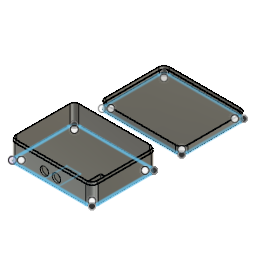
design2 (Autodesk Fusion 360 design; units mm, degrees)
Autodesk Fusion 360 part; units mm, degrees
sketch "Sketch1" plane through (0, 0, 0) normal (0, 0, 1) x (1, 0, 0)
  line L0 (10, 0) -> (170, 0)
  line L1 (180, 10) -> (180, 130)
  line L2 (170, 140) -> (10, 140)
  line L3 (0, 130) -> (0, 10)
  arc A0 (10, 140) -> (0, 130) centre (10, 130) ccw
  arc A1 (0, 10) -> (10, 0) centre (10, 10) ccw
  arc A2 (170, 0) -> (180, 10) centre (170, 10) ccw
  arc A3 (180, 130) -> (170, 140) centre (170, 130) ccw
  arc A4 (180, 130) -> (170, 140) centre (170, 130) ccw
  arc A5 (170, 0) -> (180, 10) centre (170, 10) ccw
  line L4 (-4, 130) -> (-4, 10)
  arc A6 (-4, 10) -> (10, -4) centre (10, 10) ccw
  line L5 (10, -4) -> (170, -4)
  arc A7 (170, -4) -> (184, 10) centre (170, 10) ccw
  line L6 (184, 10) -> (184, 130)
  arc A8 (184, 130) -> (170, 144) centre (170, 130) ccw
  line L7 (170, 144) -> (10, 144)
  arc A9 (10, 144) -> (-4, 130) centre (10, 130) ccw
  line L8 (-2, 130) -> (-2, 10)
  arc A10 (-2, 10) -> (10, -2) centre (10, 10) ccw
  line L9 (10, -2) -> (170, -2)
  arc A11 (170, -2) -> (182, 10) centre (170, 10) ccw
  line L10 (182, 10) -> (182, 130)
  arc A12 (182, 130) -> (170, 142) centre (170, 130) ccw
  line L11 (170, 142) -> (10, 142)
  arc A13 (10, 142) -> (-2, 130) centre (10, 130) ccw
  arc A14 (10, 142) -> (-2, 130) centre (10, 130) ccw
  arc A15 (170, -2) -> (182, 10) centre (170, 10) ccw
  line L12 (0, 130) -> (0, 10)
  line L13 (10, -4) -> (170, -4)
  arc A16 (170, 0) -> (180, 10) centre (170, 10) ccw
  line L14 (-4, 130) -> (-4, 10)
  line L15 (170, 144) -> (10, 144)
  arc A17 (184, 130) -> (170, 144) centre (170, 130) ccw
  arc A18 (10, 144) -> (-4, 130) centre (10, 130) ccw
  line L16 (10, 0) -> (170, 0)
  line L17 (-2, 130) -> (-2, 10)
  arc A19 (182, 130) -> (170, 142) centre (170, 130) ccw
  arc A20 (180, 130) -> (170, 140) centre (170, 130) ccw
  arc A21 (0, 10) -> (10, 0) centre (10, 10) ccw
  line L18 (10, -2) -> (170, -2)
  line L19 (170, 140) -> (10, 140)
  arc A22 (170, -4) -> (184, 10) centre (170, 10) ccw
  line L20 (170, 142) -> (10, 142)
  line L21 (180, 10) -> (180, 130)
  line L22 (182, 10) -> (182, 130)
  arc A23 (180, 130) -> (170, 140) centre (170, 130) ccw
  line L23 (184, 10) -> (184, 130)
  arc A24 (-4, 10) -> (10, -4) centre (10, 10) ccw
  arc A25 (10, 140) -> (0, 130) centre (10, 130) ccw
  arc A26 (170, 0) -> (180, 10) centre (170, 10) ccw
  arc A27 (-2, 10) -> (10, -2) centre (10, 10) ccw
  arc A28 (10.4205, 344.4235) -> (-1.5795, 332.4235) centre (10.4205, 332.4235) ccw
  arc A29 (170.4205, 200.4235) -> (182.4205, 212.4235) centre (170.4205, 212.4235) ccw
  line L24 (0.4205, 332.4235) -> (0.4205, 212.4235)
  line L25 (10.4205, 198.4235) -> (170.4205, 198.4235)
  arc A30 (170.4205, 202.4235) -> (180.4205, 212.4235) centre (170.4205, 212.4235) ccw
  line L26 (-3.5795, 332.4235) -> (-3.5795, 212.4235)
  line L27 (170.4205, 346.4235) -> (10.4205, 346.4235)
  arc A31 (184.4205, 332.4235) -> (170.4205, 346.4235) centre (170.4205, 332.4235) ccw
  arc A32 (10.4205, 346.4235) -> (-3.5795, 332.4235) centre (10.4205, 332.4235) ccw
  line L28 (10.4205, 202.4235) -> (170.4205, 202.4235)
  line L29 (-1.5795, 332.4235) -> (-1.5795, 212.4235)
  arc A33 (182.4205, 332.4235) -> (170.4205, 344.4235) centre (170.4205, 332.4235) ccw
  arc A34 (180.4205, 332.4235) -> (170.4205, 342.4235) centre (170.4205, 332.4235) ccw
  arc A35 (0.4205, 212.4235) -> (10.4205, 202.4235) centre (10.4205, 212.4235) ccw
  line L30 (10.4205, 200.4235) -> (170.4205, 200.4235)
  line L31 (170.4205, 342.4235) -> (10.4205, 342.4235)
  arc A36 (170.4205, 198.4235) -> (184.4205, 212.4235) centre (170.4205, 212.4235) ccw
  line L32 (170.4205, 344.4235) -> (10.4205, 344.4235)
  line L33 (180.4205, 212.4235) -> (180.4205, 332.4235)
  line L34 (182.4205, 212.4235) -> (182.4205, 332.4235)
  arc A37 (180.4205, 332.4235) -> (170.4205, 342.4235) centre (170.4205, 332.4235) ccw
  line L35 (184.4205, 212.4235) -> (184.4205, 332.4235)
  arc A38 (-3.5795, 212.4235) -> (10.4205, 198.4235) centre (10.4205, 212.4235) ccw
  arc A39 (10.4205, 342.4235) -> (0.4205, 332.4235) centre (10.4205, 332.4235) ccw
  arc A40 (170.4205, 202.4235) -> (180.4205, 212.4235) centre (170.4205, 212.4235) ccw
  arc A41 (-1.5795, 212.4235) -> (10.4205, 200.4235) centre (10.4205, 212.4235) ccw
  point P0 (180, 0)
  point P1 (180, 140)
  point P2 (0, 140)
  point P3 (180, 140)
  point P4 (0, 140)
  point P5 (180, 0)
  point P6 (180.4205, 342.4235)
  point P7 (0.4205, 342.4235)
  point P8 (0.4205, 202.4235)
  point P9 (180.4205, 202.4235)
  dimension "d1" = 140
  dimension "d2" = 180
  dimension "d3" = 10
  dimension "d4" = 4
  dimension "d5" = 2
  dimension "d6" = 4
  dimension "d7" = 2
  dimension "d8" = 140
  dimension "d9" = 180
  dimension "d10" = 10
  dimension "d11" = 4
  dimension "d12" = 2
  dimension "d13" = 140
  dimension "d14" = 180
  dimension "d15" = 10
  constraint horizontal L0
  constraint vertical L1
  constraint horizontal L2
  constraint vertical L3
  constraint coincident P4 L3
  constraint coincident P4 L2
  constraint tangent L3 A0
  constraint tangent L2 A0
  constraint tangent L3 A1
  constraint tangent L0 A1
  constraint equal A0 A1
  constraint coincident P5 L1
  constraint coincident P5 L0
  constraint tangent L1 A2
  constraint tangent L0 A2
  constraint equal A0 A2
  constraint coincident P3 L2
  constraint coincident P3 L1
  constraint tangent L2 A3
  constraint tangent L1 A3
  constraint equal A0 A3
  constraint coincident L2 A3.end
  constraint coincident L1 A3.start
  constraint tangent L2 A4
  constraint tangent L1 A4
  constraint equal A0 A4
  constraint coincident L1 A2.end
  constraint coincident L0 A2.start
  constraint tangent L1 A5
  constraint tangent L0 A5
  constraint equal A0 A5
  constraint horizontal L16
  constraint vertical L21
  constraint horizontal L19
  constraint vertical L12
  constraint coincident P4 L12
  constraint coincident P4 L19
  constraint tangent L12 A25
  constraint tangent L19 A25
  constraint tangent L12 A21
  constraint tangent L16 A21
  constraint equal A21 A25
  constraint coincident P5 L21
  constraint coincident P5 L16
  constraint tangent L21 A26
  constraint tangent L16 A26
  constraint equal A25 A26
  constraint coincident P3 L19
  constraint coincident P3 L21
  constraint tangent A20 L19
  constraint tangent A20 L21
  constraint equal A20 A25
  constraint coincident L2.start L19
  constraint coincident L1.end L21
  constraint tangent L19 A23
  constraint tangent L21 A23
  constraint equal A23 A25
  constraint coincident L1.start L21
  constraint coincident L0.end L16
  constraint tangent A16 L21
  constraint tangent A16 L16
  constraint equal A16 A25
  constraint horizontal L28
  constraint vertical L33
  constraint horizontal L31
  constraint vertical L24
  constraint coincident P7 L24
  constraint coincident P7 L31
  constraint tangent L24 A39
  constraint tangent L31 A39
  constraint tangent L24 A35
  constraint tangent L28 A35
  constraint equal A35 A39
  constraint coincident P9 L33
  constraint coincident P9 L28
  constraint tangent L33 A40
  constraint tangent L28 A40
  constraint equal A39 A40
  constraint coincident P6 L31
  constraint coincident P6 L33
  constraint tangent A34 L31
  constraint tangent A34 L33
  constraint equal A34 A39
  constraint coincident A34.end L31
  constraint coincident A34.start L33
  constraint tangent L31 A37
  constraint tangent L33 A37
  constraint equal A37 A39
  constraint coincident A30.end L33
  constraint coincident A30.start L28
  constraint tangent A30 L33
  constraint tangent A30 L28
  constraint equal A30 A39
  measures "d1" distance of P5 P3
  measures "d2" distance of P1 P4
  measures "d3" radius of A0
  measures "d8" distance of P3 P5
  measures "d9" distance of P3 P4
  measures "d10" radius of A25
  measures "d13" distance of P6 P9
  measures "d14" distance of P6 P7
  measures "d15" radius of A39
extrude "Extrude1" add sketch "Sketch1" along normal blind 4 contours L0 L1 L2 L3 A0 A1 A2 A3 A4 A5 L12 A16 L16 A20 A21 L19 L21 A23 A25 A26 | L24 A30 L28 A34 A35 L31 L33 A37 A39 A40 makes body 1 at (63.3333, 93.3333, 0) makes body 2 at (117.0871, 249.0901, 0)
extrude "Extrude2" add sketch "Sketch1" along normal blind 45 contours L8 A10 L9 A11 L10 A12 L11 A13 A14 A15 L17 A19 L18 L20 L22 A27 bodies 1
extrude "Extrude3" add sketch "Sketch1" along normal blind 40 contours L4 A6 L5 A7 L6 A8 L7 A9 L13 L14 L15 A17 A18 A22 L23 A24 bodies 1
extrude "Extrude4" add sketch "Sketch1" along normal blind 9 contours A28 A29 L29 A33 L30 L32 L34 A41 bodies 2
extrude "Extrude5" add sketch "Sketch1" along normal blind 15 contours L25 L26 L27 A31 A32 A36 L35 A38 bodies 2
sketch "Sketch2" plane through (0, 0, 0) normal (0, 1, 0) x (1, 0, 0)
  line L0 (10, -40) -> (170, -40) construction
  line L1 (90, -40) -> (90, -4) construction
  line L2 (90, -4) -> (90, -19) construction
  line L3 (76.5, -19) -> (103.5, -19)
  circle A0 centre (76.5, -19) radius 9.5
  circle A1 centre (103.5, -19) radius 9.5
  dimension "d27" = 15
  dimension "d28" = 27
  dimension "d29" = 19
  dimension "d30" = 19
  constraint horizontal L0
  constraint perpendicular L0 L1
  constraint midpoint L1 L2.end
  constraint parallel L1 L2
  constraint coincident L2.end L3
  constraint midpoint L1 L3
  measures "d27" distance of L1.end L2.end
  measures "d28" distance of L3.start L3.end
  measures "d29" diameter of A1
  measures "d30" diameter of A0
extrude "Extrude6" cut sketch "Sketch2" against normal blind 4 bodies 1
sketch "Sketch3" plane through (0, 0, 0) normal (0, 0, 1) x (1, 0, 0)
  line L0 (103.6272, 0) -> (72.8355, 0)
  line L1 (72.8355, 0) -> (72.8355, 50)
  line L2 (72.8355, 50) -> (103.6272, 50)
  line L3 (103.6272, 50) -> (103.6272, 0)
  dimension "d33" = 50
  constraint horizontal L0
  constraint vertical L1
  constraint horizontal L2
  constraint vertical L3
  measures "d33" distance of L0.end L1.end
ref_plane "WorkPlane1" through (90, 70, 24) normal (0, 0, 1) x (1, 0, 0)
sketch "Sketch4" plane through (90, 70, 24) normal (0, 0, 1) x (1, 0, 0)
  line L0 (90, -70) -> (60, -70)
  line L1 (60, -70) -> (60, -20)
  line L2 (60, -20) -> (90, -20)
  line L3 (90, -20) -> (90, -70)
  line L4 (62, -68) -> (62, -22)
  line L5 (62, -22) -> (88, -22)
  line L6 (88, -22) -> (90, -22)
  line L7 (62, -68) -> (62, -70)
  point P0 (90, -70)
  dimension "d35" = 30
  dimension "d36" = 50
  constraint horizontal L0
  constraint vertical L1
  constraint horizontal L2
  constraint vertical L3
  constraint coincident P0 L0.start
  constraint parallel L1 L4
  constraint parallel L2 L5
  constraint coincident L3 L6.end
  constraint perpendicular L3 L6
  constraint coincident L0 L7.end
  constraint perpendicular L0 L7
  measures "d35" distance of L1.end L2.end
  measures "d36" distance of L0.end L1.end
extrude "Extrude7" add sketch "Sketch4" against normal blind 20 contours L0 L1 L2 L3 L4 L5 L6 L7 bodies 1
